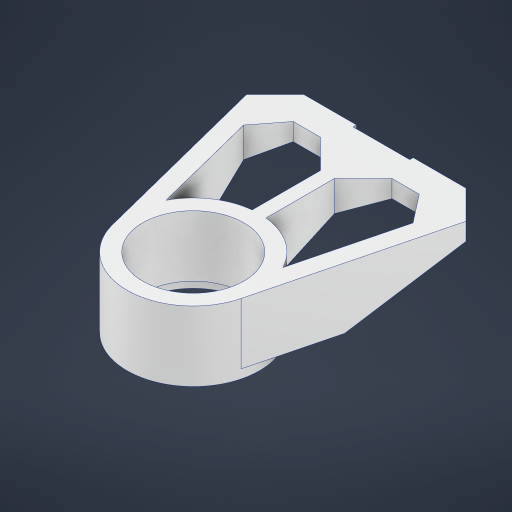
# Autodesk Inventor part: KrovatkaShatunPods
Saved by Autodesk Inventor 2024 (Build 280153000, 153)
## iProperties
Created: 2023-12-22
Part Number: KrovatkaShatunPods
Material: Aluminum 6061
Document SubType Name: Modeling
Designer: KirikDK
Mass: 3341.8 g
Surface Area: 1685.96 cm^2
Volume: 1237.7 cm^3
Density: 2.7 g/cm^3
Appearance: Aluminum - Flat
Author: KirikDK
Autodesk Inventor part; units mm, degrees
ref_plane "YZ Plane" through (0, 0, 0) normal (1, 0, 0) x (0, 1, 0)
ref_plane "XZ Plane" through (0, 0, 0) normal (0, 1, 0) x (-1, 0, 0)
ref_plane "XY Plane" through (0, 0, 0) normal (0, 0, 1) x (1, 0, 0)
sketch "Sketch1" plane through (0, 0, 0) normal (0, 1, 0) x (-1, 0, 0)
  circle A0 centre (0, 0) radius 62.05
  circle A1 centre (0, 0) radius 76
  dimension "d0" = 124.1
  constraints: 2 centre point, 2 coincident
  measures "d0" diameter of A0
extrude "Extrusion1" add sketch "Sketch1" along normal blind 10
sketch "Sketch2" plane through (0, 10, 0) normal (0, 1, 0) x (1, 0, 0)
  circle A0 centre (0, 0) radius 76 projected
  circle A1 centre (0, 0) radius 62.05 projected
  line L0 (-76, 0) -> (76, 0)
  line L1 (76, 0) -> (76, 220)
  line L2 (76, 220) -> (-76, 220)
  line L3 (-76, 220) -> (-76, 0)
  line L4 (-126, 220) -> (126, 220)
  line L5 (126, 220) -> (126, 187)
  line L6 (126, 187) -> (-126, 187)
  line L7 (-126, 187) -> (-126, 220)
  line L8 (126, 187) -> (73.6534, -18.7397)
  circle A2 centre (0, 0) radius 76 projected
  line L9 (-126, 187) -> (-73.6534, -18.7397)
  point P0 (-73.6534, -18.7397)
  point P1 (73.6534, -18.7397)
  dimension "d3" = 220
  dimension "d4" = 50
  dimension "d5" = 50
  dimension "d15" = 33
  dimension "d16" = 76
  dimension "d17" = 76
  dimension "d18" = 126
  constraints: 20 end point, 4 parallel, 2 horizontal, 2 perpendicular, 2 point on circle, 2 tangent, 1 midpoint, 1 point on line, 2 other
  measures "d3" distance of L2.end L0.start
  measures "d4" distance between parallel lines of L7 L3
  measures "d5" distance between parallel lines of L1 L5
  measures "d15" distance of L6.end L4.start
  measures "d16" distance from line of point (0, 0) L3
  measures "d17" distance from line of point (0, 0) L1
  measures "d18" distance from line of point (0, 0) L5
extrude "Extrusion2" add sketch "Sketch2" along normal blind 70
sketch "Sketch3" plane through (126, 10, -187) normal (1, 0, 0) x (0, 0, -1)
  line L0 (39, 50) -> (0, 50)
  line L1 (0, 0) -> (0, 70) projected
  line L2 (0, 50) -> (-111, 0)
  line L3 (-205.7397, 0) -> (0, 0) projected
  line L4 (39, 50) -> (39, 0)
  line L5 (39, 0) -> (-111, 0)
  line L6 (0, 70) -> (33, 70) projected
  point P0 (-187, -10)
  dimension "d10" = 20
  constraints: 8 end point, 2 point on line, 1 horizontal, 1 perpendicular, 1 vertical
  measures "d10" distance between parallel lines of L6 L0
extrude "Extrusion3" cut sketch "Sketch3" against normal blind 300
sketch "Sketch4" plane through (0, 10, 0) normal (0, -1, 0) x (1, 0, 0)
  circle A0 centre (0, 0) radius 58
  line L0 (-97.7581, -76) -> (97.7581, -76) projected
  circle A1 centre (0, 0) radius 76
  line L1 (126, -220) -> (-126, -220) projected
  line L2 (126, -187) -> (126, -220) projected
  line L3 (126, -187) -> (-126, -187) projected
  line L4 (-126, -220) -> (-126, -187) projected
  line L5 (97.7581, -76) -> (126, -187) projected
  line L6 (0, -76) -> (97.7581, -76) projected
  line L7 (-97.7581, -76) -> (0, -76) projected
  line L8 (-126, -187) -> (-97.7581, -76) projected
  line L9 (126, -187) -> (-126, -187) projected
  line L10 (0, -76) -> (97.7581, -76) projected
  line L11 (73.6534, 18.7397) -> (97.7581, -76) projected
  arc A2 (0, -76) -> (73.6534, 18.7397) centre (0, 0) ccw projected
  line L12 (-97.7581, -76) -> (0, -76) projected
  arc A3 (-73.6534, 18.7397) -> (0, -76) centre (0, 0) ccw projected
  line L13 (-97.7581, -76) -> (-73.6534, 18.7397) projected
  line L14 (64.6258, -26.8898) -> (109.6331, -203.7836)
  line L15 (-65.3309, -29.6614) -> (-109.9518, -205.0363)
  line L16 (8, -74) -> (-8, -74)
  line L17 (-8, -74) -> (-8, -228)
  line L18 (-8, -228) -> (8, -228)
  line L19 (8, -228) -> (8, -74)
  line L20 (0, -76) -> (97.7581, -76) projected
  circle A4 centre (0, 0) radius 62.05 projected
  line L21 (73.6534, 18.7397) -> (97.7581, -76) projected
  arc A5 (0, -76) -> (73.6534, 18.7397) centre (0, 0) ccw projected
  line L22 (-97.7581, -76) -> (0, -76) projected
  circle A6 centre (0, 0) radius 62.05 projected
  arc A7 (-73.6534, 18.7397) -> (0, -76) centre (0, 0) ccw projected
  line L23 (-97.7581, -76) -> (-73.6534, 18.7397) projected
  point P0 (-8, -75.5778)
  point P1 (-66.9402, -35.9863)
  point P2 (-105.3628, -187)
  point P3 (-8, -187)
  point P4 (8, -187)
  point P5 (105.3628, -187)
  point P6 (66.9402, -35.9863)
  point P7 (8, -75.5778)
  dimension "d11" = 20
  dimension "d12" = 20
  constraints: 12 end point, 4 parallel, 2 coincident, 1 centre point, 1 horizontal, 1 perpendicular, 3 other
  measures "d11" distance between parallel lines of L5 L14
  measures "d12" distance between parallel lines of L8 L15
extrude "Extrusion5" cut sketch "Sketch4" against normal blind 300 contours A0 | L15 A1 L17 L0 | L0 L17 L3 L15 | L19 A1 L14 L0 | L0 L14 L3 L19
chamfer "Chamfer1" distance 33 angle 45 6 edges at (-126, 70, -220) (126, 70, -220) (105.3628, 70, -187) (-105.3628, 70, -187) (8, 70, -187) (-8, 70, -187)
sketch "Sketch7" plane through (93, 60, -220) normal (0, 0, -1) x (-1, 0, 0)
  line L0 (0, 20) -> (186, 20) projected
  line L1 (0, 0) -> (186, 0) projected
  line L2 (125.5, 20) -> (60.5, 20)
  line L3 (60.5, 20) -> (60.5, 0)
  line L4 (60.5, 0) -> (125.5, 0)
  line L5 (125.5, 0) -> (125.5, 20)
  line L6 (186, 20) -> (186, 0) projected
  line L7 (0, 0) -> (0, 20) projected
  point P0 (93, -60)
  point P1 (125.5, 0)
  point P2 (60.5, 20)
  dimension "d24" = 65
  dimension "d25" = 60.5
  dimension "d26" = 60.5
  constraints: 8 end point, 2 parallel, 2 point on line, 1 horizontal, 1 perpendicular
  measures "d24" distance between parallel lines of L3 L5
  measures "d25" distance between parallel lines of L6 L5
  measures "d26" distance between parallel lines of L3 L7
extrude "Extrusion6" cut sketch "Sketch7" against normal blind 4 contours L0 L5 L1 L3
body "Solid1"
